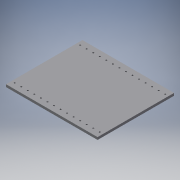
# Autodesk Inventor part: MCPlate2
Saved by Autodesk Inventor 2016 (Build 200138000, 138)
## iProperties
Created: 2015-09-04
Part Number: MCPlate2
Material: Generic
Document SubType Name: Modeling
Designer: Tim
Density: 1 g/cm^3
Appearance: Default
Author: Tim
Autodesk Inventor part; units mm, degrees
ref_plane "YZ Plane" through (0, 0, 0) normal (1, 0, 0) x (0, 1, 0)
ref_plane "XZ Plane" through (0, 0, 0) normal (0, 1, 0) x (-1, 0, 0)
ref_plane "XY Plane" through (0, 0, 0) normal (0, 0, 1) x (1, 0, 0)
sketch "Sketch1" plane through (0, 0, 0) normal (0, 0, 1) x (1, 0, 0)
  line L0 (-112, -93.5) -> (112, -93.5)
  line L1 (112, -93.5) -> (112, 93.5)
  line L2 (112, 93.5) -> (-112, 93.5)
  line L3 (-112, 93.5) -> (-112, -93.5)
  line L4 (-112, -93.5) -> (112, 93.5) construction
  line L5 (112, -93.5) -> (-112, 93.5) construction
  line L6 (-104, -80) -> (104, 80) construction
  line L7 (104, -80) -> (-104, 80) construction
  circle A0 centre (-104, 80) radius 1.85
  circle A1 centre (-104, -80) radius 1.85
  circle A2 centre (104, -80) radius 1.85
  circle A3 centre (104, 80) radius 1.85
  circle A4 centre (-88, 80) radius 1.85 projected
  circle A5 centre (-72, 80) radius 1.85 projected
  circle A6 centre (-56, 80) radius 1.85 projected
  circle A7 centre (-40, 80) radius 1.85 projected
  circle A8 centre (-24, 80) radius 1.85 projected
  circle A9 centre (-8, 80) radius 1.85 projected
  circle A10 centre (8, 80) radius 1.85 projected
  circle A11 centre (24, 80) radius 1.85 projected
  circle A12 centre (40, 80) radius 1.85 projected
  circle A13 centre (56, 80) radius 1.85 projected
  circle A14 centre (72, 80) radius 1.85 projected
  circle A15 centre (88, 80) radius 1.85 projected
  circle A16 centre (-88, -80) radius 1.85 projected
  circle A17 centre (-72, -80) radius 1.85 projected
  circle A18 centre (-56, -80) radius 1.85 projected
  circle A19 centre (-40, -80) radius 1.85 projected
  circle A20 centre (-24, -80) radius 1.85 projected
  circle A21 centre (-8, -80) radius 1.85 projected
  circle A22 centre (8, -80) radius 1.85 projected
  circle A23 centre (24, -80) radius 1.85 projected
  circle A24 centre (40, -80) radius 1.85 projected
  circle A25 centre (56, -80) radius 1.85 projected
  circle A26 centre (72, -80) radius 1.85 projected
  circle A27 centre (88, -80) radius 1.85 projected
  circle A28 centre (8, -64) radius 1.85 projected
  circle A29 centre (8, -48) radius 1.85 projected
  circle A30 centre (8, -32) radius 1.85 projected
  circle A31 centre (40, -64) radius 1.85 projected
  circle A32 centre (40, -32) radius 1.85 projected
  circle A33 centre (40, -48) radius 1.85 projected
  circle A34 centre (8, -16) radius 1.85 projected
  circle A35 centre (8, 0) radius 1.85 projected
  circle A36 centre (40, -16) radius 1.85 projected
  circle A37 centre (40, 0) radius 1.85 projected
  circle A38 centre (40, 16) radius 1.85 projected
  circle A39 centre (40, 32) radius 1.85 projected
  circle A40 centre (40, 48) radius 1.85 projected
  circle A41 centre (40, 64) radius 1.85 projected
  circle A42 centre (8, 48) radius 1.85 projected
  circle A43 centre (8, 16) radius 1.85 projected
  circle A44 centre (8, 32) radius 1.85 projected
  circle A45 centre (8, 64) radius 1.85 projected
  circle A46 centre (72, -64) radius 1.85 projected
  circle A47 centre (72, -48) radius 1.85 projected
  circle A48 centre (72, -32) radius 1.85 projected
  circle A49 centre (72, 0) radius 1.85 projected
  circle A50 centre (72, -16) radius 1.85 projected
  circle A51 centre (72, 16) radius 1.85 projected
  circle A52 centre (72, 32) radius 1.85 projected
  circle A53 centre (72, 48) radius 1.85 projected
  circle A54 centre (72, 64) radius 1.85 projected
  circle A55 centre (104, 64) radius 1.85 projected
  circle A56 centre (104, 48) radius 1.85 projected
  circle A57 centre (104, 32) radius 1.85 projected
  circle A58 centre (104, 16) radius 1.85 projected
  circle A59 centre (104, 0) radius 1.85 projected
  circle A60 centre (104, -16) radius 1.85 projected
  circle A61 centre (104, -32) radius 1.85 projected
  circle A62 centre (104, -48) radius 1.85 projected
  circle A63 centre (104, -64) radius 1.85 projected
  circle A64 centre (-104, -64) radius 1.85 projected
  circle A65 centre (-72, -64) radius 1.85 projected
  circle A66 centre (-104, -48) radius 1.85 projected
  circle A67 centre (-72, -48) radius 1.85 projected
  circle A68 centre (-104, -32) radius 1.85 projected
  circle A69 centre (-72, -32) radius 1.85 projected
  circle A70 centre (-104, -16) radius 1.85 projected
  circle A71 centre (-72, -16) radius 1.85 projected
  circle A72 centre (-104, 0) radius 1.85 projected
  circle A73 centre (-72, 0) radius 1.85 projected
  circle A74 centre (-104, 16) radius 1.85 projected
  circle A75 centre (-72, 16) radius 1.85 projected
  circle A76 centre (-104, 32) radius 1.85 projected
  circle A77 centre (-72, 32) radius 1.85 projected
  circle A78 centre (-72, 48) radius 1.85 projected
  circle A79 centre (-104, 48) radius 1.85 projected
  circle A80 centre (-104, 64) radius 1.85 projected
  circle A81 centre (-72, 64) radius 1.85 projected
  circle A82 centre (-40, -64) radius 1.85 projected
  circle A83 centre (-8, -64) radius 1.85 projected
  circle A84 centre (-40, -48) radius 1.85 projected
  circle A85 centre (-8, -48) radius 1.85 projected
  circle A86 centre (-40, -32) radius 1.85 projected
  circle A87 centre (-8, -32) radius 1.85 projected
  circle A88 centre (-40, -16) radius 1.85 projected
  circle A89 centre (-8, -16) radius 1.85 projected
  circle A90 centre (-40, 0) radius 1.85 projected
  circle A91 centre (-8, 0) radius 1.85 projected
  circle A92 centre (-40, 16) radius 1.85 projected
  circle A93 centre (-8, 16) radius 1.85 projected
  circle A94 centre (-40, 32) radius 1.85 projected
  circle A95 centre (-8, 32) radius 1.85 projected
  circle A96 centre (-40, 48) radius 1.85 projected
  circle A97 centre (-8, 48) radius 1.85 projected
  circle A98 centre (-40, 64) radius 1.85 projected
  circle A99 centre (-8, 64) radius 1.85 projected
  point P0 (0, 0)
  dimension "d0" = 224
  dimension "d1" = 187
  dimension "d16" = 3.7
  dimension "d17" = 3.7
  dimension "d18" = 3.7
  dimension "d19" = 3.7
  dimension "d20" = 160
  dimension "d21" = 208
  constraints: 16 end point, 4 centre point, 4 coincident, 3 midpoint, 2 parallel, 1 horizontal, 1 perpendicular
  measures "d0" distance of L2.end L1.end
  measures "d1" distance of L1.end L0.end
  measures "d16" diameter of A0
  measures "d17" diameter of A1
  measures "d18" diameter of A2
  measures "d19" diameter of A3
  measures "d20" distance of L6.start L7.end
  measures "d21" distance of L7.start L6.start
extrude "Extrusion8" add sketch "Sketch1" along normal blind 6
body "Solid8"
